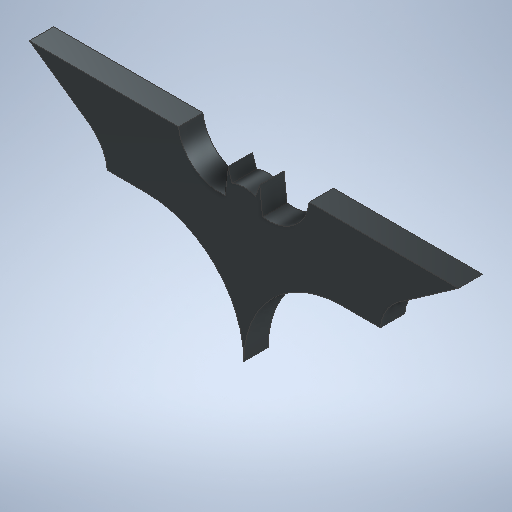
# Autodesk Inventor part: Batarang
Saved by Autodesk Inventor 2025.2 (Build 292293000, 293)
## iProperties
Created: 2025-05-11
Part Number: Batarang
Material: Generic
Document SubType Name: Modeling
Designer: Miguel
Density: 1 g/cm^3
Appearance: Default
Author: Miguel
Autodesk Inventor part; units mm, degrees
ref_plane "YZ Plane" through (0, 0, 0) normal (1, 0, 0) x (0, 1, 0)
ref_plane "XZ Plane" through (0, 0, 0) normal (0, 1, 0) x (-1, 0, 0)
ref_plane "XY Plane" through (0, 0, 0) normal (0, 0, 1) x (1, 0, 0)
sketch "Sketch1" plane through (0, 0, 0) normal (0, 0, 1) x (1, 0, 0)
  line L0 (0, 110.8966) -> (0, -110.8966) construction
  line L1 (-205.6207, 0) -> (205.6207, 0) construction
  line L2 (-67, 75) -> (-220, 75)
  line L3 (-220, 75) -> (-158.9525, 32.2541)
  line L4 (-140, 0) -> (-100, 0)
  arc A0 (-140, 0) -> (-158.9525, 32.2541) centre (-184.7635, -4.6077) ccw
  arc A1 (0, -100) -> (-100, 0) centre (-100, -100) ccw
  arc A2 (0, 55) -> (-12, 52.4955) centre (0, 25) ccw
  line L5 (-12, 52.4955) -> (-16.3057, 65)
  line L6 (-16.3057, 65) -> (-19.1435, 38)
  arc A3 (-67, 75) -> (-19.1435, 38) centre (-25.2476, 79.5541) ccw
  line L7 (205.6207, 0) -> (-205.6207, 0) construction
  line L8 (67, 75) -> (220, 75)
  line L9 (220, 75) -> (158.9525, 32.2541)
  line L10 (140, 0) -> (100, 0)
  arc A4 (158.9525, 32.2541) -> (140, 0) centre (184.7635, -4.6077) ccw
  arc A5 (100, 0) -> (0, -100) centre (100, -100) ccw
  arc A6 (12, 52.4955) -> (0, 55) centre (0, 25) ccw
  line L11 (12, 52.4955) -> (16.3057, 65)
  line L12 (16.3057, 65) -> (19.1435, 38)
  arc A7 (19.1435, 38) -> (67, 75) centre (25.2476, 79.5541) ccw
  point P0 (0, 0)
  point P1 (0, 0)
  dimension "d1" = 67
  dimension "d2" = 220
  dimension "d3" = 35
  dimension "d4" = 45
  dimension "d5" = 140
  dimension "d7" = 75
  dimension "d8" = 100
  dimension "d9" = 100
  dimension "d10" = 30
  dimension "d11" = 50
  dimension "d12" = 12
  dimension "d13" = 10
  dimension "d14" = 37
  dimension "d15" = 25
  dimension "d21" = 42
  dimension "d23" = 84
  constraints: 26 end point, 16 point on circle, 13 symmetric about line, 8 centre point, 7 point on line, 2 midpoint, 2 tangent, 1 coincident, 1 horizontal, 1 perpendicular, 1 vertical, 4 other
  measures "d1" distance from line of L2.start L0
  measures "d2" distance from line of L0 L2.end
  measures "d3" angle of L2 L3
  measures "d4" radius of A0
  measures "d5" distance from line of L0 L4.start
  measures "d7" distance from line of L4.end L2
  measures "d8" distance from line of L1 A1.start
  measures "d9" radius of A1
  measures "d10" radius of A2
  measures "d11" distance from line of L2 A2.centre
  measures "d12" distance from line of L0 L5.start
  measures "d13" distance from line of L2 L5.end
  measures "d14" distance from line of L2 L6.end
  measures "d15" angle of L6 L5
  measures "d21" radius of A3
  measures "d23" angle of L6 L2
extrude "Extrusion1" add sketch "Sketch1" along normal blind 25
body "Solid1"
